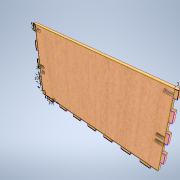
# Autodesk Inventor part: DoosjeVoorkant
Saved by Autodesk Inventor 2021 (Build 250183000, 183)
## iProperties
Created: 2021-03-11
Part Number: DoosjeVoorkant
Material: Wood (Cherry)
Document SubType Name: Modeling
Designer: ZiweZhang
Density: 0.63 g/cm^3
Appearance: Cherry - Natural Low Gloss
Author: ZiweZhang
Autodesk Inventor part; units mm, degrees
ref_plane "YZ Plane" through (0, 0, 0) normal (1, 0, 0) x (0, 1, 0)
ref_plane "XZ Plane" through (0, 0, 0) normal (0, 1, 0) x (-1, 0, 0)
ref_plane "XY Plane" through (0, 0, 0) normal (0, 0, 1) x (1, 0, 0)
sketch "Sketch1" plane through (0, 0, 0) normal (0, 0, 1) x (1, 0, 0)
  line L0 (0, 0) -> (99, 0)
  line L1 (99, 0) -> (99, 77)
  line L2 (99, 77) -> (0, 77)
  line L3 (0, 77) -> (0, 0)
  dimension "d0" = 99
  dimension "d1" = 77
  constraints: 8 end point, 2 parallel, 1 horizontal, 1 perpendicular
  measures "d0" distance of L2.end L1.end
  measures "d1" distance of L1.end L0.end
extrude "Extrusion1" add sketch "Sketch1" along normal blind 3
sketch "Sketch2" plane through (0, 0, 3) normal (0, 0, 1) x (1, 0, 0)
  line L0 (99, 77) -> (0, 77) projected
  line L1 (0, 0) -> (99, 0) projected
  line L2 (0, 77) -> (99, 77)
  line L3 (99, 77) -> (99, 0)
  line L4 (99, 0) -> (0, 0)
  line L5 (0, 0) -> (0, 77)
  line L6 (0, 77) -> (0, 0) projected
  line L7 (0, 10) -> (-3, 10)
  line L8 (-3, 10) -> (-3, 20)
  line L9 (-3, 20) -> (0, 20)
  line L10 (-3, 40) -> (0, 40)
  line L11 (-3, 30) -> (-3, 40)
  line L12 (0, 30) -> (-3, 30)
  line L13 (-3, 60) -> (0, 60)
  line L14 (-3, 50) -> (-3, 60)
  line L15 (0, 50) -> (-3, 50)
  line L16 (99, 77) -> (0, 77) projected
  line L17 (0, 77) -> (-3, 77)
  line L18 (-3, 77) -> (-3, 70)
  line L19 (-3, 70) -> (0, 70)
  line L20 (99, 0) -> (99, 77) projected
  line L21 (99, 77) -> (102, 77)
  line L22 (102, 77) -> (102, 70)
  line L23 (102, 70) -> (99, 70)
  line L24 (99, 0) -> (99, 77) projected
  line L25 (99, 60) -> (102, 60)
  line L26 (102, 60) -> (102, 50)
  line L27 (102, 50) -> (99, 50)
  line L28 (99, 40) -> (102, 40)
  line L29 (102, 40) -> (102, 30)
  line L30 (102, 30) -> (99, 30)
  line L31 (99, 20) -> (102, 20)
  line L32 (102, 20) -> (102, 10)
  line L33 (102, 10) -> (99, 10)
  line L34 (99, 10) -> (99, -3)
  line L35 (99, -3) -> (93.25, -3)
  line L36 (93.25, -3) -> (93.25, 0)
  line L37 (93.25, 0) -> (75.75, 0)
  line L38 (75.75, 0) -> (75.75, -3)
  line L39 (75.75, -3) -> (58.25, -3)
  line L40 (58.25, -3) -> (58.25, 0)
  line L41 (58.25, 0) -> (40.75, 0)
  line L42 (40.75, 0) -> (40.75, -3)
  line L43 (40.75, -3) -> (23.25, -3)
  line L44 (23.25, -3) -> (23.25, 0)
  line L45 (23.25, 0) -> (5.75, 0)
  line L46 (5.75, 0) -> (5.75, -3)
  line L47 (5.75, -3) -> (0, -3)
  line L48 (0, -3) -> (0, 0)
  point P0 (99, 30)
  point P1 (99, 20)
  point P2 (99, 10)
  point P3 (23.25, 0)
  point P4 (58.25, 0)
  point P5 (93.25, 0)
  dimension "d13" = 3
  dimension "d14" = 10
  dimension "d17" = 20
  dimension "d22" = 3
  dimension "d23" = 7
  dimension "d24" = 3
  dimension "d48" = 13
  dimension "d49" = 5.75
  dimension "d50" = 17.5
  dimension "d51" = 17.5
  dimension "d52" = 17.5
  dimension "d53" = 17.5
  dimension "d54" = 17.5
  dimension "d55" = 5.75
  constraints: 84 end point, 20 perpendicular, 13 point on line, 5 horizontal, 2 parallel, 2 vertical, 31 other
  measures "d13" distance of L7.start L7.end
  measures "d14" distance of L7.end L8.end
  measures "d17" distance of L8.end L10.start
  measures "d22" distance of L0.end L17.end
  measures "d23" distance of L17.end L18.end
  measures "d24" distance of L0.start L21.end
  measures "d48" distance of L33.end L34.end
  measures "d49" distance of L34.end L35.end
  measures "d50" distance of L36.end L37.end
  measures "d51" distance of L38.end L39.end
  measures "d52" distance of L40.end L41.end
  measures "d53" distance of L42.end L43.end
  measures "d54" distance of L44.end L45.end
  measures "d55" distance of L46.end L47.end
extrude "Extrusion2" add sketch "Sketch2" against normal blind 3 contours L21 L22 L23 L3 | L5 L19 L18 L17 | L25 L26 L27 L3 | L5 L15 L14 L13 | L28 L29 L30 L3 | L5 L12 L11 L10 | L31 L32 L33 L3 | L5 L7 L8 L9 | L34 L35 L36 L1 | L1 L46 L47 L48 | L38 L39 L40 L1 | L1 L42 L43 L44
sketch "Sketch3" plane through (0, 0, 3) normal (0, 0, 1) x (1, 0, 0)
  line L0 (0, 73.9) -> (7, 73.9)
  line L1 (7, 73.9) -> (7, 70.9)
  line L2 (7, 70.9) -> (0, 70.9)
  line L3 (0, 70.9) -> (0, 73.9)
  line L4 (92, 73.9) -> (99, 73.9)
  line L5 (99, 73.9) -> (99, 70.9)
  line L6 (99, 70.9) -> (92, 70.9)
  line L7 (92, 70.9) -> (92, 73.9)
  line L8 (0, 35.9) -> (7, 35.9)
  line L9 (7, 35.9) -> (7, 32.9)
  line L10 (7, 32.9) -> (0, 32.9)
  line L11 (0, 32.9) -> (0, 35.9)
  line L12 (92, 35.9) -> (99, 35.9)
  line L13 (99, 35.9) -> (99, 32.9)
  line L14 (99, 32.9) -> (92, 32.9)
  line L15 (92, 32.9) -> (92, 35.9)
  line L16 (7, 29.9) -> (7, 26.9)
  line L17 (7, 26.9) -> (0, 26.9)
  line L18 (0, 26.9) -> (0, 29.9)
  line L19 (0, 29.9) -> (7, 29.9)
  line L20 (99, 35.9) -> (99, 32.9)
  line L21 (99, 32.9) -> (92, 32.9)
  line L22 (92, 32.9) -> (92, 35.9)
  line L23 (92, 35.9) -> (99, 35.9)
  line L24 (99, 29.9) -> (99, 26.9)
  line L25 (99, 26.9) -> (92, 26.9)
  line L26 (92, 26.9) -> (92, 29.9)
  line L27 (92, 29.9) -> (99, 29.9)
  line L28 (-3, 77) -> (102, 77) projected
  line L29 (99, 20) -> (99, 30) projected
  point P0 (0, 0)
  dimension "d27" = 7
  dimension "d28" = 3
  dimension "d31" = 92
  dimension "d34" = 38
  dimension "d41" = 6
  dimension "d44" = 92
  dimension "d47" = 3.1
  constraints: 56 end point, 4 collinear, 3 horizontal, 3 perpendicular, 2 vertical, 44 other
  measures "d27" distance of L0.start L0.end
  measures "d28" distance of L0.end L1.end
  measures "d31" distance of L0.start L4.start
  measures "d34" distance of L0.start L8.start
  measures "d41" distance of L10.end L17.end
  measures "d44" distance of L10.end L21.end
  measures "d47" distance between parallel lines of L4 L28
extrude "Extrusion3" cut sketch "Sketch3" against normal through all
body "Solid1"
